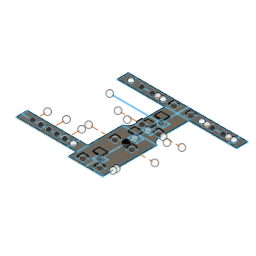
finger flat v4 (Autodesk Fusion 360 design; units mm, degrees)
Autodesk Fusion 360 part; units mm, degrees
note: some values were not read from the file. Chosen so that the rebuilt part matches the saved one: which bodies a step acts on; which face or edge a step refers to. Set by a fixed rule: which sketch regions a step uses.
sketch "Sketch2" plane through (0, 0, 0) normal (0, 0, 1) x (1, 0, 0)
  circle A0 centre (0, 0) radius 11.5
  line L0 (0, 0) -> (0, -11.5)
  line L1 (9.9593, -5.75) -> (-9.9593, -5.75)
  line L2 (9.9593, -5.75) -> (-9.9593, -5.75)
  arc A1 (-9.9593, -5.75) -> (9.9593, -5.75) centre (0, 0) ccw
  dimension "d6" = 23
  constraint coincident A0.centre L0.start
  constraint coincident A0 L0.end
  constraint vertical L0
  constraint coincident A0 L1.start
  constraint coincident A0 L1.end
  constraint coincident L0.end A1
  measures "d6" diameter of A0
sketch "Sketch3" plane through (0, 0, 0) normal (0, 0, 1) x (1, 0, 0)
  line L0 (0, -37.5) -> (0, -12.5)
  line L1 (0, -12.5) -> (0, -7.5)
  line L2 (0, -7.5) -> (0, 7.5)
  line L3 (0, 7.5) -> (0, 12.5)
  line L4 (0, 12.5) -> (0, 32.5)
  line L5 (0, 32.5) -> (0, 57.5)
  line L6 (0, 57.5) -> (48, 57.5)
  line L7 (48, 57.5) -> (48, 47.5)
  line L8 (48, 47.5) -> (0, 47.5)
  line L9 (0, 47.5) -> (-48, 47.5)
  line L10 (-48, 57.5) -> (0, 57.5)
  line L11 (0, 32.5) -> (-47.7177, 32.5)
  line L12 (-24, -25) -> (-72, -25)
  line L13 (-72, -25) -> (-72, -20)
  line L14 (-72, -20) -> (-24, -20)
  line L15 (-24, -20) -> (-24, -30)
  line L16 (-24, -30) -> (-72, -30)
  line L17 (-72, -30) -> (-72, -20)
  line L18 (15.8003, -25) -> (15.8003, -28)
  line L19 (-72, -30) -> (-62, -30) construction
  line L20 (-62, -30) -> (-62, -11.1593) construction
  line L21 (-62, -30) -> (-47, -30) construction
  line L22 (-47, -30) -> (-32, -30) construction
  line L23 (-47, -30) -> (-47, -8.6093) construction
  line L24 (-32, -30) -> (-32, -9.4061) construction
  circle A0 centre (-62, -25) radius 2.5
  circle A1 centre (-47, -25) radius 2.5
  circle A2 centre (-32, -25) radius 2.5
  line L25 (-11, 22.5) -> (-11, 25.5)
  line L26 (-11, 19.5) -> (-11, 22.5)
  line L27 (12, 22.5) -> (11, 22.5)
  line L28 (11, 22.5) -> (11, 25.5)
  line L29 (11, 19.5) -> (11, 22.5)
  line L30 (48, 52.5) -> (38, 52.5) construction
  circle A3 centre (-38, 52.5) radius 2.5
  circle A4 centre (38, 52.5) radius 2.5
  line L31 (-38, 52.5) -> (-28, 52.5)
  line L32 (38, 52.5) -> (28, 52.5)
  circle A5 centre (28, 52.5) radius 2.5
  circle A6 centre (-28, 52.5) radius 2.5
  line L33 (-15.8, -12.5) -> (-15.8, 12.5)
  line L34 (11, 25.5) -> (11, 47.5)
  line L35 (-11, 25.5) -> (-11, 47.5)
  line L36 (-15.8, -12.5) -> (-15.8, -37.5)
  line L37 (15.8, 10) -> (15.8003, -22)
  line L38 (-24, -20) -> (-15.8, -20)
  line L39 (-24, -30) -> (-15.8, -30)
  line L40 (-15.8, -37.5) -> (15.8003, -37.5)
  line L41 (15.8003, -22) -> (15.8003, -37.5)
  circle A7 centre (0, -25) radius 2
  line L42 (-2, -25) -> (-3, -25)
  line L43 (-3, -25) -> (-3, -22)
  line L44 (-3, -22) -> (5, -22)
  line L45 (5, -22) -> (5, -28)
  line L46 (5, -28) -> (-3, -28)
  line L47 (-3, -28) -> (-3, -25)
  line L48 (-34.5, -25) -> (-39.5, -25)
  line L49 (-49.5, -25) -> (-54.5, -25)
  circle A8 centre (-39.5, -25) radius 2.5
  circle A9 centre (-54.5, -25) radius 2.5
  line L50 (-15.8, 12.5) -> (15.8, 12.5003)
  line L51 (15.8, 12.5003) -> (15.8, 10)
  arc A10 (-15.8, 12.5) -> (-11, 19.5) centre (-18.5042, 19.5) ccw
  arc A11 (11, 19.5) -> (15.8, 12.5003) centre (18.5037, 19.5) ccw
  circle A12 centre (23, 52.5) radius 2.5 construction
  circle A13 centre (18, 52.5) radius 2.5
  circle A14 centre (-23, 52.5) radius 2.5 construction
  circle A15 centre (-18, 52.5) radius 2.5
  circle A16 centre (43, 52.5) radius 2.5 construction
  circle A17 centre (48, 52.5) radius 2.5
  circle A18 centre (-48, 52.5) radius 2.5
  circle A19 centre (0, 32.5) radius 2
  circle A20 centre (0, 20.5) radius 2
  circle A21 centre (0, 8) radius 2
  line L52 (-2, 8) -> (-3, 8)
  line L53 (-3, 8) -> (-3, 11)
  line L54 (-3, 11) -> (5, 11)
  line L55 (5, 11) -> (5, 5)
  line L56 (5, 5) -> (-3, 5)
  line L57 (-3, 8) -> (-3, 5)
  line L58 (-2, 20.5) -> (-3, 20.5)
  line L59 (-3, 20.5) -> (-3, 23.5)
  line L60 (-3, 23.5) -> (5, 23.5)
  line L61 (5, 23.5) -> (5, 17.5)
  line L62 (5, 17.5) -> (-3, 17.5)
  line L63 (-3, 17.5) -> (-3, 20.5)
  line L64 (-2, 32.5) -> (-3, 32.5)
  line L65 (-3, 32.5) -> (-3, 35.5)
  line L66 (-3, 35.5) -> (5, 35.5)
  line L67 (5, 35.5) -> (5, 29.5)
  line L68 (5, 29.5) -> (-3, 29.5)
  line L69 (-3, 29.5) -> (-3, 32.5)
  line L70 (55.5, 57.5) -> (55.5, 47.5)
  line L71 (48, 47.5) -> (55.5, 47.5)
  line L72 (55.5, 57.5) -> (48, 57.5)
  line L73 (-55.5, 52.5) -> (-55.5, 57.5)
  line L74 (-55.5, 57.5) -> (-48, 57.5)
  line L75 (-48, 47.5) -> (-55.5, 47.5)
  line L76 (-55.5, 47.5) -> (-55.5, 52.5)
  line L77 (15.8003, -37.5) -> (7.8003, -37.5)
  line L78 (7.8003, -37.5) -> (7.8003, 57.5) construction
  line L79 (-15.8, -37.5) -> (-7.8, -37.5) construction
  line L80 (-7.8, -37.5) -> (-7.8, 57.5) construction
  line L81 (7.8003, -37.5) -> (7.8003, -32.5) construction
  line L82 (-7.8, -37.5) -> (-7.8, -32.5) construction
  line L83 (10.3003, -30) -> (5.3003, -30)
  line L84 (5.3003, -30) -> (5.3003, -35)
  line L85 (5.3003, -35) -> (10.3003, -35)
  line L86 (10.3003, -35) -> (10.3003, -30)
  line L87 (10.3003, -30) -> (5.3003, -35) construction
  line L88 (5.3003, -30) -> (10.3003, -35) construction
  line L89 (-5.3, -30) -> (-10.3, -30)
  line L90 (-10.3, -30) -> (-10.3, -35)
  line L91 (-10.3, -35) -> (-5.3, -35)
  line L92 (-5.3, -35) -> (-5.3, -30)
  line L93 (-5.3, -30) -> (-10.3, -35) construction
  line L94 (-10.3, -30) -> (-5.3, -35) construction
  line L95 (0, -37.5) -> (0, -2.5) construction
  line L96 (0, -2.5) -> (29.2324, -2.4997) construction
  line L97 (0, -2.5) -> (-32.3166, -2.4998) construction
  line L98 (-5.3, 0) -> (-10.3, 0)
  line L99 (-10.3, 0) -> (-10.3, -5)
  line L100 (-10.3, -5) -> (-5.3, -5)
  line L101 (-5.3, -5) -> (-5.3, 0)
  line L102 (-5.3, 0) -> (-10.3, -5) construction
  line L103 (-10.3, 0) -> (-5.3, -5) construction
  line L104 (10.3003, 0.0001) -> (5.3003, 0.0001)
  line L105 (5.3003, 0.0001) -> (5.3003, -4.9999)
  line L106 (5.3003, -4.9999) -> (10.3003, -4.9999)
  line L107 (10.3003, -4.9999) -> (10.3003, 0.0001)
  line L108 (10.3003, 0.0001) -> (5.3003, -4.9999) construction
  line L109 (5.3003, 0.0001) -> (10.3003, -4.9999) construction
  line L110 (0, -37.5) -> (0, 22.5) construction
  line L111 (0, 22.5) -> (29.4799, 22.5) construction
  line L112 (0, 22.5) -> (-30.0065, 22.5) construction
  line L113 (-5.3, 25) -> (-10.3, 25)
  line L114 (-10.3, 25) -> (-10.3, 20)
  line L115 (-10.3, 20) -> (-5.3, 20)
  line L116 (-5.3, 20) -> (-5.3, 25)
  line L117 (-5.3, 25) -> (-10.3, 20) construction
  line L118 (-10.3, 25) -> (-5.3, 20) construction
  line L119 (10.3003, 25) -> (5.3003, 25)
  line L120 (5.3003, 25) -> (5.3003, 20)
  line L121 (5.3003, 20) -> (10.3003, 20)
  line L122 (10.3003, 20) -> (10.3003, 25)
  line L123 (10.3003, 25) -> (5.3003, 20) construction
  line L124 (5.3003, 25) -> (10.3003, 20) construction
  line L125 (0, 47.5) -> (0, 52.5)
  line L126 (0, 52.5) -> (7.8003, 52.5) construction
  line L127 (0, 52.5) -> (-7.8, 52.5) construction
  line L128 (-5.3, 55) -> (-10.3, 55)
  line L129 (-10.3, 55) -> (-10.3, 50)
  line L130 (-10.3, 50) -> (-5.3, 50)
  line L131 (-5.3, 50) -> (-5.3, 55)
  line L132 (-5.3, 55) -> (-10.3, 50) construction
  line L133 (-10.3, 55) -> (-5.3, 50) construction
  line L134 (10.3003, 55) -> (5.3003, 55)
  line L135 (5.3003, 55) -> (5.3003, 50)
  line L136 (5.3003, 50) -> (10.3003, 50)
  line L137 (10.3003, 50) -> (10.3003, 55)
  line L138 (10.3003, 55) -> (5.3003, 50) construction
  line L139 (5.3003, 55) -> (10.3003, 50) construction
  point P0 (7.8003, -32.5)
  point P1 (-7.8, -32.5)
  point P2 (-7.8, -2.5)
  point P3 (7.8003, -2.4999)
  point P4 (-7.8, 22.5)
  point P5 (7.8003, 22.5)
  point P6 (-7.8, 52.5)
  point P7 (7.8003, 52.5)
  dimension "d9" = 25
  dimension "d10" = 5
  dimension "d11" = 15
  dimension "d12" = 5
  dimension "d13" = 20
  dimension "d14" = 25
  dimension "d15" = 48
  dimension "d16" = 10
  dimension "d17" = 48
  dimension "d18" = 10
  dimension "d20" = 48
  dimension "d22" = 5
  dimension "d23" = 10
  dimension "d28" = 10
  dimension "d29" = 15
  dimension "d30" = 15
  dimension "d31" = 5
  dimension "d32" = 5
  dimension "d33" = 5
  dimension "d40" = 3
  dimension "d43" = 1
  dimension "d44" = 3
  dimension "d49" = 10
  dimension "d53" = 5
  dimension "d55" = 5
  dimension "d57" = 10
  dimension "d58" = 10
  dimension "d59" = 5
  dimension "d60" = 5
  dimension "d75" = 4
  dimension "d76" = 1
  dimension "d77" = 3
  dimension "d78" = 8
  dimension "d79" = 6
  dimension "d80" = 5
  dimension "d81" = 5
  dimension "d82" = 5
  dimension "d83" = 5
  dimension "d84" = 5
  dimension "d85" = 5
  dimension "d86" = 5
  dimension "d87" = 5
  dimension "d88" = 5
  dimension "d89" = 5
  dimension "d91" = 5
  dimension "d94" = 4
  dimension "d97" = 4
  dimension "d99" = 4
  dimension "d100" = 1
  dimension "d101" = 3
  dimension "d102" = 8
  dimension "d103" = 6
  dimension "d104" = 1
  dimension "d105" = 3
  dimension "d106" = 8
  dimension "d107" = 6
  dimension "d108" = 1
  dimension "d109" = 3
  dimension "d110" = 8
  dimension "d111" = 6
  dimension "d122" = 8
  dimension "d123" = 8
  dimension "d124" = 5
  dimension "d125" = 5
  dimension "d126" = 5
  dimension "d127" = 5
  dimension "d128" = 5
  dimension "d129" = 5
  dimension "d130" = 35
  dimension "d131" = 5
  dimension "d132" = 5
  dimension "d133" = 5
  dimension "d134" = 5
  dimension "d135" = 60
  dimension "d136" = 5
  dimension "d137" = 5
  dimension "d138" = 5
  dimension "d139" = 5
  dimension "d140" = 5
  dimension "d141" = 5
  dimension "d142" = 5
  dimension "d143" = 5
  dimension "d144" = 5
  constraint perpendicular L5 L6
  constraint perpendicular L6 L7
  constraint coincident L5 L8.end
  constraint perpendicular L5 L8
  constraint perpendicular L5 L9
  constraint perpendicular L5 L11
  constraint perpendicular L12 L13
  constraint horizontal L14
  constraint vertical L15
  constraint horizontal L16
  constraint vertical L17
  constraint coincident L16 L19.end
  constraint perpendicular L16 L20
  constraint coincident L16 L21.end
  constraint parallel L16 L22
  constraint perpendicular L21 L23
  constraint perpendicular L22 L24
  constraint coincident L12 A0.centre
  constraint coincident L20 A0.centre
  constraint coincident L23 A1.centre
  constraint coincident L12 A1.centre
  constraint coincident L24 A2.centre
  constraint coincident L12 A2.centre
  constraint perpendicular L26 L27
  constraint perpendicular L27 L28
  constraint perpendicular L27 L29
  constraint midpoint L7 L30.start
  constraint coincident A3.centre L31.start
  constraint coincident L30.end A4.centre
  constraint coincident L32.end A5.centre
  constraint coincident L31.end A6.centre
  constraint coincident L8 L34.end
  constraint perpendicular L8 L34
  constraint coincident L9 L35.end
  constraint perpendicular L9 L35
  constraint coincident L36 L38.end
  constraint perpendicular L36 L38
  constraint coincident L36 L39.end
  constraint perpendicular L36 L39
  constraint perpendicular L40 L41
  constraint midpoint L0 A7.centre
  constraint coincident A7 L42.start
  constraint perpendicular L0 L42
  constraint perpendicular L42 L43
  constraint perpendicular L0 L44
  constraint perpendicular L42 L45
  constraint perpendicular L0 L46
  constraint perpendicular L42 L47
  constraint coincident L12 L48.start
  constraint coincident A2 L48.start
  constraint parallel L12 L48
  constraint coincident A1 L49.start
  constraint coincident L12 L49.end
  constraint perpendicular L23 L49
  constraint coincident L48.end A8.centre
  constraint coincident L49.end A9.centre
  constraint perpendicular L37 L50
  constraint vertical L51
  constraint tangent L26 A10
  constraint tangent L29 A11
  constraint coincident L4.end L5.start
  constraint coincident A21 L52.start
  constraint perpendicular L3 L52
  constraint perpendicular L52 L53
  constraint perpendicular L3 L54
  constraint perpendicular L54 L55
  constraint perpendicular L2 L56
  constraint perpendicular L56 L57
  constraint coincident A20 L58.start
  constraint perpendicular L4 L58
  constraint perpendicular L58 L59
  constraint perpendicular L4 L60
  constraint perpendicular L58 L61
  constraint perpendicular L4 L62
  constraint perpendicular L58 L63
  constraint coincident A19 L64.start
  constraint coincident L11 L64.start
  constraint perpendicular L63 L64
  constraint perpendicular L64 L65
  constraint perpendicular L5 L66
  constraint perpendicular L66 L67
  constraint perpendicular L4 L68
  constraint perpendicular L64 L69
  constraint perpendicular L70 L71
  constraint perpendicular L7 L72
  constraint perpendicular L10 L73
  constraint perpendicular L73 L75
  constraint coincident L40 L77.end
  constraint perpendicular L0 L77
  constraint coincident L6 L78.end
  constraint perpendicular L6 L78
  constraint coincident L40 L79.end
  constraint perpendicular L36 L79
  constraint coincident L10 L80.end
  constraint perpendicular L10 L80
  constraint coincident L78 P0
  constraint perpendicular L77 L81
  constraint coincident L80 P1
  constraint horizontal L83
  constraint perpendicular L83 L84
  constraint parallel L83 L85
  constraint parallel L84 L86
  constraint coincident L87 P0
  constraint coincident L88 P0
  constraint coincident P0 L81.end
  constraint horizontal L89
  constraint perpendicular L89 L90
  constraint parallel L89 L91
  constraint parallel L90 L92
  constraint coincident L93 P1
  constraint coincident L94 P1
  constraint coincident P1 L82.end
  constraint coincident L2 L95.end
  constraint parallel L2 L95
  constraint perpendicular L37 L96
  constraint horizontal L98
  constraint perpendicular L98 L99
  constraint parallel L98 L100
  constraint parallel L99 L101
  constraint coincident L102 P2
  constraint coincident L103 P2
  constraint coincident L97 P2
  constraint coincident L80 P2
  constraint horizontal L104
  constraint perpendicular L104 L105
  constraint parallel L104 L106
  constraint parallel L105 L107
  constraint coincident L108 P3
  constraint coincident L109 P3
  constraint coincident L78 P3
  constraint coincident L96 P3
  constraint midpoint L4 L110.end
  constraint tangent A20 L111
  constraint perpendicular L61 L111
  constraint tangent A20 L112
  constraint perpendicular L59 L112
  constraint horizontal L113
  constraint perpendicular L113 L114
  constraint parallel L113 L115
  constraint parallel L114 L116
  constraint coincident L117 P4
  constraint coincident L118 P4
  constraint coincident L80 P4
  constraint coincident L112 P4
  constraint horizontal L119
  constraint perpendicular L119 L120
  constraint parallel L119 L121
  constraint parallel L120 L122
  constraint coincident L123 P5
  constraint coincident L124 P5
  constraint coincident L78 P5
  constraint coincident L111 P5
  constraint coincident L5 L125.end
  constraint coincident L78 P7
  constraint perpendicular L78 L126
  constraint coincident L80 P6
  constraint perpendicular L80 L127
  constraint horizontal L128
  constraint perpendicular L128 L129
  constraint parallel L128 L130
  constraint parallel L129 L131
  constraint coincident L132 P6
  constraint coincident L133 P6
  constraint coincident P6 L127.end
  constraint horizontal L134
  constraint perpendicular L134 L135
  constraint parallel L134 L136
  constraint parallel L135 L137
  constraint coincident L138 P7
  constraint coincident L139 P7
  constraint coincident P7 L126.end
  measures "d9" distance of L0.start L0.end
  measures "d10" distance of L0.end L1.end
  measures "d11" distance of L1.end L2.end
  measures "d12" distance of L2.end L3.end
  measures "d13" distance of L3.end L4.end
  measures "d14" distance of L4.end L5.end
  measures "d15" distance of L5.end L6.end
  measures "d16" distance of L6.end L7.end
  measures "d17" distance of L8.end L9.end
  measures "d18" distance of L9.end L10.start
  measures "d20" distance of L12.start L12.end
  measures "d22" distance of L12.end L13.end
  measures "d23" distance of L13.end L16.end
  measures "d28" distance of L16.end L19.end
  measures "d29" distance of L19.end L21.end
  measures "d30" distance of L21.end L22.end
  measures "d31" diameter of A0
  measures "d32" diameter of A1
  measures "d33" diameter of A2
  measures "d40" distance of L25.start L25.end
  measures "d43" distance of L27.start L27.end
  measures "d44" distance of L27.end L28.end
  measures "d49" distance of L30.start L30.end
  measures "d53" diameter of A3
  measures "d55" diameter of A4
  measures "d57" distance of A3.centre L31.end
  measures "d58" distance of L30.end L32.end
  measures "d59" diameter of A5
  measures "d60" diameter of A6
  measures "d75" diameter of A7
  measures "d76" distance of L42.start L42.end
  measures "d77" distance of L42.end L43.end
  measures "d78" distance of L43.end L44.end
  measures "d79" distance of L44.end L45.end
  measures "d80" distance of L48.start L48.end
  measures "d81" distance of L49.start L49.end
  measures "d82" diameter of A8
  measures "d83" diameter of A9
  measures "d84" diameter of A12
  measures "d85" diameter of A13
  measures "d86" diameter of A14
  measures "d87" diameter of A15
  measures "d88" diameter of A16
  measures "d89" diameter of A17
  measures "d91" diameter of A18
  measures "d94" diameter of A19
  measures "d97" diameter of A20
  measures "d99" diameter of A21
  measures "d100" distance of L52.start L52.end
  measures "d101" distance of L52.end L53.end
  measures "d102" distance of L53.end L54.end
  measures "d103" distance of L54.end L55.end
  measures "d104" distance of L58.start L58.end
  measures "d105" distance of L58.end L59.end
  measures "d106" distance of L59.end L60.end
  measures "d107" distance of L60.end L61.end
  measures "d108" distance of L64.start L64.end
  measures "d109" distance of L64.end L65.end
  measures "d110" distance of L65.end L66.end
  measures "d111" distance of L66.end L67.end
  measures "d122" distance of L40.end L77.end
  measures "d123" distance of L36.end L79.end
  measures "d124" distance of L77.end P0
  measures "d125" distance of L79.end P1
  measures "d126" distance of L84.end L85.end
  measures "d127" distance of L83.end L84.end
  measures "d128" distance of L90.end L91.end
  measures "d129" distance of L89.end L90.end
  measures "d130" distance of L0.start L95.end
  measures "d131" distance of L99.end L100.end
  measures "d132" distance of L98.end L99.end
  measures "d133" distance of L105.end L106.end
  measures "d134" distance of L104.end L105.end
  measures "d135" distance of L0.start L110.end
  measures "d136" distance of L114.end L115.end
  measures "d137" distance of L113.end L114.end
  measures "d138" distance of L120.end L121.end
  measures "d139" distance of L119.end L120.end
  measures "d140" distance of L8.end L125.end
  measures "d141" distance of L129.end L130.end
  measures "d142" distance of L128.end L129.end
  measures "d143" distance of L135.end L136.end
  measures "d144" distance of L134.end L135.end
extrude "Extrude8" add sketch "Sketch3" along normal blind 6.4 contours L0 A7 L42 L46 L47 | L0 A7 L44 L45 L46 | L0 A7 | L0 A7 | L0 A7 L42 L43 L44 | L2 A21 L52 L56 L57 | L2 L3 A21 L54 L55 L56 | L3 A21 L52 L53 L54 | L4 A20 L58 L62 L63 | L4 A20 L60 L61 L62 | L2 L3 A21 | L2 L3 A21 | L4 A20 | L4 A20 | L4 A20 L58 L59 L60 | L5 L11 A19 L64 L65 L66 | L4 L11 A19 L64 L68 L69 | L4 L5 A19 L66 L67 L68 | L5 L11 A19 | L4 L11 A19 | L4 L5 A19 makes body 1 at (-0.3333, 11, 2.1333) makes body 2 at (-0.3333, 23.5, 2.1333) makes body 3 at (-0.3333, -22, 2.1333) makes body 4 at (2.3333, 29.5, 2.1333)
extrude "Extrude9" add sketch "Sketch3" along normal blind 0.4 contours L0 L1 L2 L3 L33 L36 L40 L43 L44 L46 L47 L50 L53 L54 L56 L57 | L0 L1 L2 L3 L18 L37 L40 L41 L44 L45 L46 L50 L51 L54 L55 L56 L77 | L15 L36 L38 L39 | L12 L15 L16 L17 A0 A1 A2 L48 L49 A8 A9 | L12 L13 L14 L15 L17 A0 A1 A2 L48 L49 A8 A9 | L4 L11 L25 L26 L35 L50 A10 L59 L60 L62 L63 L68 L69 | L4 L5 L8 L28 L29 L34 L50 A11 L60 L61 L62 L66 L67 L68 | L5 L9 L11 L35 L65 L66 | L5 L9 L10 L73 L74 L75 L76 L125 | L5 L6 L7 L8 A17 L125 | L7 A17 L70 L71 L72 | L83 L84 L85 L86 | L89 L90 L91 L92 | L98 L99 L100 L101 | L104 L105 L106 L107 | L113 L114 L115 L116 | L119 L120 L121 L122 | L128 L129 L130 L131 | L134 L135 L136 L137 bodies 1 2 3 4
extrude "Extrude10" cut sketch "Sketch3" along normal blind 5.4 contours L0 A7 L42 L46 L47 | L0 A7 L44 L45 L46 | L0 A7 L42 L43 L44 | L2 A21 L52 L56 L57 | L2 L3 A21 L54 L55 L56 | L3 A21 L52 L53 L54 | L4 A20 L58 L62 L63 | L4 A20 L60 L61 L62 | L4 A20 L58 L59 L60 | L5 L11 A19 L64 L65 L66 | L4 L11 A19 L64 L68 L69 | L4 L5 A19 L66 L67 L68 bodies 1 makes body 5 at (1.9901, 32.6991, 1.8) makes body 6 at (1.9901, -24.8009, 1.8) makes body 7 at (1.9901, 20.6991, 1.8) makes body 8 at (1.9901, 7.8009, 3.6)
extrude "Extrude11" add sketch "Sketch3" along normal blind 0.4 contours L0 A7 L42 L46 L47 | L0 A7 L44 L45 L46 | L0 A7 L42 L43 L44 | L2 A21 L52 L56 L57 | L2 L3 A21 L54 L55 L56 | L3 A21 L52 L53 L54 | L4 A20 L58 L62 L63 | L4 A20 L60 L61 L62 | L4 A20 L58 L59 L60 | L5 L11 A19 L64 L65 L66 | L4 L11 A19 L64 L68 L69 | L4 L5 A19 L66 L67 L68 bodies 1 5 6 7 8
extrude "Extrude12" add sketch "Sketch3" along normal blind 3.4 contours L83 L84 L85 L86 | L89 L90 L91 L92 | L98 L99 L100 L101 | L104 L105 L106 L107 | L113 L114 L115 L116 | L119 L120 L121 L122 | L128 L129 L130 L131 | L134 L135 L136 L137 bodies 1
extrude "Extrude13" cut 8 faces at (-8.6333, 53.3333, 3.4) (6.967, 53.3333, 3.4) (-8.6333, 23.3333, 3.4) (6.967, 23.3333, 3.4) (-8.6333, -1.6666, 3.4) (6.967, -1.6666, 3.4) (6.967, -33.3333, 3.4) (-8.6333, -33.3333, 3.4) along direction (0, 0, -1) blind 1 on bodies 1 bodies 1
hole "Hole1" at (7.8003, -35, 1.4) direction (0, 1, 0) diameter 0.6 end through all bodies 1
hole "Hole2" at (-7.8, -35, 1.4) direction (0, 1, 0) diameter 0.6 end through all bodies 1
